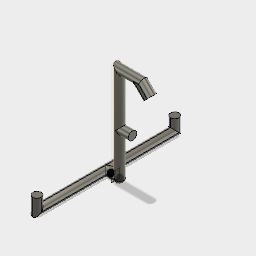
pegboard-hook-002 (Autodesk Fusion 360 design; units mm, degrees)
Autodesk Fusion 360 part; units mm, degrees
sketch "スケッチ3" plane through (0, 0, 0) normal (0, 1, 0) x (1, 0, 0)
  line L0 (5, -5) -> (10, -5)
  line L1 (10, -5) -> (10, -10)
  line L2 (10, -10) -> (5, -10)
  line L3 (5, -10) -> (5, -5)
  line L4 (-10, 0) -> (-5, 0)
  line L5 (-5, 0) -> (-5, 60)
  line L6 (-5, 60) -> (-10, 60)
  line L7 (-10, 60) -> (-10, 0)
  line L8 (10, 10) -> (10, 5)
  line L9 (10, 5) -> (17, 5)
  line L10 (17, 10) -> (10, 10)
  line L11 (-5, 55) -> (-10, 55)
  line L12 (-10, 55) -> (-10, 0)
  line L13 (-10, 0) -> (-5, 0)
  line L14 (-5, 0) -> (-5, 55)
  line L15 (5, 0) -> (10, 0)
  line L16 (10, 0) -> (10, 60)
  line L17 (10, 60) -> (5, 60)
  line L18 (5, 60) -> (5, 0)
  line L19 (17, 5) -> (17, 10)
  line L20 (5, 0) -> (10, 0)
  line L21 (10, 0) -> (10, 60)
  line L22 (10, 60) -> (5, 60)
  line L23 (5, 60) -> (5, 0)
  line L24 (22, 60) -> (5, 60)
  line L25 (5, 60) -> (5, 5)
  line L26 (5, 5) -> (-3, 5)
  line L27 (-3, 5) -> (-3, 0)
  line L28 (-3, 0) -> (10, 0)
  line L29 (10, 0) -> (10, 25)
  line L30 (10, 25) -> (15, 25)
  line L31 (15, 25) -> (15, 30)
  line L32 (15, 30) -> (10, 30)
  line L33 (10, 30) -> (10, 55)
  line L34 (10, 55) -> (17, 55)
  line L35 (17, 55) -> (22.6569, 49.3431)
  line L36 (22.6569, 49.3431) -> (27.6569, 54.3431)
  line L37 (27.6569, 54.3431) -> (22, 60)
  line L38 (-17, 55) -> (-10, 55)
  line L39 (-10, 55) -> (-10, 30)
  line L40 (-10, 30) -> (-15, 30)
  line L41 (-15, 30) -> (-15, 25)
  line L42 (-15, 25) -> (-10, 25)
  line L43 (-10, 25) -> (-10, 0)
  line L44 (-10, 0) -> (3, 0)
  line L45 (3, 0) -> (3, 5)
  line L46 (3, 5) -> (-5, 5)
  line L47 (-5, 5) -> (-5, 60)
  line L48 (-5, 60) -> (-22, 60)
  line L49 (-22, 60) -> (-27.6569, 54.3431)
  line L50 (-27.6569, 54.3431) -> (-22.6569, 49.3431)
  line L51 (-22.6569, 49.3431) -> (-17, 55)
  line L52 (-5, 10) -> (-5, 5)
  line L53 (-5, 5) -> (-2, 5)
  line L54 (-2, 5) -> (-2, -35)
  line L55 (-2, -35) -> (3, -35)
  line L56 (3, -35) -> (3, 50)
  line L57 (3, 50) -> (-2, 50)
  line L58 (-2, 50) -> (-2, 10)
  line L59 (-2, 10) -> (-5, 10)
  line L60 (3, 45) -> (-2, 45)
  line L61 (-2, 45) -> (-2, 10)
  line L62 (-2, 10) -> (-5, 10)
  line L63 (-5, 10) -> (-5, 5)
  line L64 (-5, 5) -> (-2, 5)
  line L65 (-2, 5) -> (-2, -35)
  line L66 (-2, -35) -> (3, -35)
  line L67 (3, -35) -> (3, 45)
  point P0 (-2, 5)
  dimension "d4" = 5
  dimension "d5" = 5
  measures "d4" distance of L0 L2
  measures "d5" distance of L1 L3
  measures "d17" distance of L11.end
extrude "押し出し2" add sketch "スケッチ3" along normal blind 60 contours L0 L1 L2 L3
sketch "スケッチ4" plane through (10, 0, 0) normal (1, 0, 0) x (0, 0, -1)
  line L0 (-10, 0) -> (-5, 0)
  line L1 (-5, 0) -> (-5, 60)
  line L2 (-5, 60) -> (-10, 60)
  line L3 (-10, 60) -> (-10, 0)
  line L4 (-10, 60) -> (-5, 60)
  line L5 (-5, 60) -> (-5, 55)
  line L6 (-5, 55) -> (-10, 55)
  line L7 (-10, 55) -> (-10, 60)
  dimension "d10" = 5
  measures "d10" distance of L4 L6
extrude "押し出し4" add sketch "スケッチ4" along normal blind 12 contours L1 L2 L3 L4 L5 L6 L7
chamfer "面取り1" distance 5 angle 45 1 edges at (22, 55, 7.5)
extrude "押し出し9" add 2 faces at (22, 59.9997, 8.3333) (20.3337, 58.3327, 6.6667) along direction (0.707107, -0.707107, 0) blind 8
sketch "スケッチ5" plane through (0, 55, 0) normal (0, -1, 0) x (1, 0, 0)
  line L0 (10, 10) -> (10, 5)
  line L1 (10, 5) -> (17, 5)
  line L2 (17, 10) -> (10, 10)
  line L3 (17, 10) -> (12, 10)
  line L4 (12, 10) -> (12, 5)
  line L5 (12, 5) -> (17, 5)
  line L6 (17, 5) -> (17, 10)
  line L7 (17, 5) -> (17, 10)
  dimension "d13" = 5
  measures "d13" distance of L4 L6
sketch "スケッチ7" plane through (10, 0, 0) normal (1, 0, 0) x (0, 0, -1)
  line L0 (-5, 55) -> (-10, 55)
  line L1 (-10, 55) -> (-10, 0)
  line L2 (-10, 0) -> (-5, 0)
  line L3 (-5, 0) -> (-5, 55)
  line L4 (-10, 30) -> (-5, 30)
  line L5 (-5, 30) -> (-5, 25)
  line L6 (-5, 25) -> (-10, 25)
  line L7 (-10, 25) -> (-10, 30)
  dimension "d17" = 25
  dimension "d18" = 5
  measures "d17" distance of L0.end L4
  measures "d18" distance of L4 L6
extrude "押し出し6" add sketch "スケッチ7" along normal blind 5 contours L1 L3 L4 L5 L6 L7
sketch "スケッチ8" plane through (5, 0, 0) normal (-1, 0, 0) x (0, 0, 1)
  line L0 (5, 0) -> (10, 0)
  line L1 (10, 0) -> (10, 60)
  line L2 (10, 60) -> (5, 60)
  line L3 (5, 60) -> (5, 0)
  line L4 (5, 0) -> (10, 0)
  line L5 (10, 0) -> (10, 5)
  line L6 (10, 5) -> (5, 5)
  line L7 (5, 5) -> (5, 0)
  dimension "d21" = 5
  measures "d21" distance of L4 L6
sketch "スケッチ14" plane through (5, 0, 0) normal (-1, 0, 0) x (0, 0, 1)
  line L0 (5, 0) -> (10, 0)
  line L1 (10, 0) -> (10, 60)
  line L2 (10, 60) -> (5, 60)
  line L3 (5, 60) -> (5, 0)
  line L4 (5, 0) -> (10, 0)
  line L5 (10, 0) -> (10, 5)
  line L6 (10, 5) -> (5, 5)
  line L7 (5, 5) -> (5, 0)
  dimension "d51" = 5
  measures "d51" distance of L4 L6
extrude "押し出し15" add sketch "スケッチ14" along normal blind 8 contours L0 L1 L3 L4 L5 L6 L7
sketch "スケッチ15" plane through (0, 0, 10) normal (0, 0, 1) x (1, 0, 0)
  line L0 (22, 60) -> (5, 60)
  line L1 (5, 60) -> (5, 5)
  line L2 (5, 5) -> (-3, 5)
  line L3 (-3, 5) -> (-3, 0)
  line L4 (-3, 0) -> (10, 0)
  line L5 (10, 0) -> (10, 25)
  line L6 (10, 25) -> (15, 25)
  line L7 (15, 25) -> (15, 30)
  line L8 (15, 30) -> (10, 30)
  line L9 (10, 30) -> (10, 55)
  line L10 (10, 55) -> (17, 55)
  line L11 (17, 55) -> (22.6569, 49.3431)
  line L12 (22.6569, 49.3431) -> (27.6569, 54.3431)
  line L13 (27.6569, 54.3431) -> (22, 60)
  line L14 (-3, 0) -> (2, 0)
  line L15 (2, 0) -> (2, 5)
  line L16 (2, 5) -> (-3, 5)
  line L17 (-3, 5) -> (-3, 0)
  dimension "d56" = 5
  measures "d56" distance of L15 L17
extrude "押し出し16" add sketch "スケッチ15" along normal blind 40 contours L2 L3 L4 L14 L15 L16 L17
sketch "スケッチ16" plane through (0, 0, 5) normal (0, 0, -1) x (-1, 0, 0)
  line L0 (-17, 55) -> (-10, 55)
  line L1 (-10, 55) -> (-10, 30)
  line L2 (-10, 30) -> (-15, 30)
  line L3 (-15, 30) -> (-15, 25)
  line L4 (-15, 25) -> (-10, 25)
  line L5 (-10, 25) -> (-10, 0)
  line L6 (-10, 0) -> (3, 0)
  line L7 (3, 0) -> (3, 5)
  line L8 (3, 5) -> (-5, 5)
  line L9 (-5, 5) -> (-5, 60)
  line L10 (-5, 60) -> (-22, 60)
  line L11 (-22, 60) -> (-27.6569, 54.3431)
  line L12 (-27.6569, 54.3431) -> (-22.6569, 49.3431)
  line L13 (-22.6569, 49.3431) -> (-17, 55)
  line L14 (3, 0) -> (-2, 0)
  line L15 (-2, 0) -> (-2, 5)
  line L16 (-2, 5) -> (3, 5)
  line L17 (3, 5) -> (3, 0)
  point P0 (-2, 5)
extrude "押し出し17" add sketch "スケッチ16" along normal blind 40 contours L6 L7 L8 L14 L15 L16 L17
sketch "スケッチ17" plane through (0, 5, 0) normal (0, 1, 0) x (-1, 0, 0)
  line L0 (-5, 10) -> (-5, 5)
  line L1 (-5, 5) -> (-2, 5)
  line L2 (-2, 5) -> (-2, -35)
  line L3 (-2, -35) -> (3, -35)
  line L4 (3, -35) -> (3, 50)
  line L5 (3, 50) -> (-2, 50)
  line L6 (-2, 50) -> (-2, 10)
  line L7 (-2, 10) -> (-5, 10)
  line L8 (3, 50) -> (-2, 50)
  line L9 (-2, 50) -> (-2, 45)
  line L10 (-2, 45) -> (3, 45)
  line L11 (3, 45) -> (3, 50)
  dimension "d61" = 5
  measures "d61" distance of L8 L10
extrude "押し出し18" add sketch "スケッチ17" along normal blind 5 contours L4 L5 L6 L8 L9 L10 L11
sketch "スケッチ18" plane through (0, 5, 0) normal (0, 1, 0) x (-1, 0, 0)
  line L0 (3, 45) -> (-2, 45)
  line L1 (-2, 45) -> (-2, 10)
  line L2 (-2, 10) -> (-5, 10)
  line L3 (-5, 10) -> (-5, 5)
  line L4 (-5, 5) -> (-2, 5)
  line L5 (-2, 5) -> (-2, -35)
  line L6 (-2, -35) -> (3, -35)
  line L7 (3, -35) -> (3, 45)
  line L8 (3, -35) -> (-2, -35)
  line L9 (-2, -35) -> (-2, -30)
  line L10 (-2, -30) -> (3, -30)
  line L11 (3, -30) -> (3, -35)
  dimension "d64" = 5
  measures "d64" distance of L8 L10
extrude "押し出し19" add sketch "スケッチ18" along normal blind 5 contours L5 L6 L7 L8 L9 L10 L11
fillet "フィレット9" radius 2.5 18 edges at (13.5, 60, 10) (13.5, 60, 5) (24.8284, 57.1716, 5) (24.8284, 57.1716, 10) (19.8284, 52.1716, 10) (19.8284, 52.1716, 5) (13.5, 55, 5) (13.5, 55, 10) (5, 32.5, 10) (5, 32.5, 5) (10, 42.5, 10) (10, 42.5, 5) (12.5, 30, 5) (12.5, 30, 10) (12.5, 25, 10) (12.5, 25, 5) (10, 12.5, 10) (10, 12.5, 5)
fillet "フィレット11" radius 2.5 19 edges at (4.75, 5, 10) (4.75, 5, 5) (2, 5, -12.5) (2, 5, 27.5) (-3, 5, 7.5) (-3, 0, 7.5) (2, 0, 30) (2, 5, 50) (-3, 5, 50) (2, 7.5, 45) (-3, 7.5, 45) (-3, 7.5, -30) (2, 7.5, -30) (-3, 5, -35) (2, 5, -35) (2, 0, -15) (4.75, 0, 5) (10, 0, 7.5) (4.75, 0, 10)
